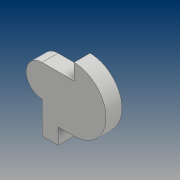
# Autodesk Inventor part: 44 (16853.982 mm^3)
Saved by Autodesk Inventor 2018 (Build 220112000, 112)
## iProperties
Created: 2020-09-18
Part Number: 44 (16853.982 mm^3)
Material: 一般
Document SubType Name: Modeling
Designer: 88697
Density: 1 g/cm^3
Appearance: 預設
Author: 88697
Autodesk Inventor part; units mm, degrees
ref_plane "YZ Plane" through (0, 0, 0) normal (1, 0, 0) x (0, 1, 0)
ref_plane "XZ Plane" through (0, 0, 0) normal (0, 1, 0) x (-1, 0, 0)
ref_plane "XY Plane" through (0, 0, 0) normal (0, 0, 1) x (1, 0, 0)
sketch "草圖1" plane through (0, 0, 0) normal (0, 1, 0) x (-1, 0, 0)
  arc A0 (0, -10) -> (0, 10) centre (0, 0) ccw
  line L0 (-20, -20) -> (-10, -20)
  line L1 (-10, -20) -> (-10, -10)
  line L2 (-10, -10) -> (0, -10)
  line L3 (-20, 20) -> (-20, 10)
  line L4 (-20, 10) -> (0, 10)
  arc A1 (-20, 20) -> (-20, -20) centre (-20, 0) ccw
  dimension "d0" = 20
  dimension "d2" = 20
  dimension "d3" = 0
  dimension "d4" = 10
  dimension "d5" = 10
  dimension "d6" = 10
  dimension "d7" = 20
  dimension "d8" = 20
  constraints: 10 end point, 4 point on circle, 3 perpendicular, 2 centre point, 1 coincident, 1 horizontal, 1 tangent, 1 vertical
  measures "d0" diameter of A0
  measures "d2" distance of point (0, 0) A1.centre
  measures "d3" vertical distance of point (0, 0) A1.centre
  measures "d4" distance of L0.start L0.end
  measures "d5" distance of L0.end L1.end
  measures "d6" distance of L3.start L3.end
  measures "d7" distance from line of point (0, 0) L3
  measures "d8" radius of A1
extrude "擠出1" add sketch "草圖1" along normal blind 10
sketch "草圖3" plane through (10, 0, -20) normal (-1, 0, 0) x (0, 0, 1)
  line L0 (10, 0) -> (0, 0) projected
  line L1 (10, 0) -> (-10, 0)
  line L2 (-10, 0) -> (-10, 30)
  line L3 (-10, 30) -> (10, 10)
  line L4 (10, 0) -> (10, 10) projected
  line L5 (10, 10) -> (10, 0)
  point P0 (20, 0)
  dimension "d11" = 20
  dimension "d12" = 30
  dimension "d13" = 0
  constraints: 8 end point, 1 collinear, 1 horizontal, 1 perpendicular
  measures "d11" distance between parallel lines of L4 L2
  measures "d12" distance of L1.end L2.end
  measures "d13" distance of L4.end L3.end
extrude "擠出2" add sketch "草圖3" along normal blind 10
